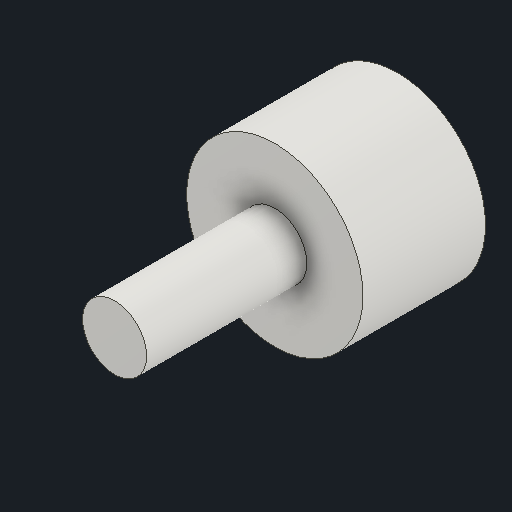
# Autodesk Inventor part: Flat Pulley1
Saved by Autodesk Inventor 2024.2 (Build 282272000, 272)
## iProperties
CustomPartVersion: 1
Created: 2024-03-22
Part Number: Flat Pulley1
Material: Steel
Document SubType Name: Modeling
Designer: LightStore
Density: 7.85 g/cm^3
Appearance: Steel
d3: 0.000 mm
d4: 0.000 mm
Author: LightStore
Autodesk Inventor part; units mm, degrees
ref_plane "YZ Plane" through (0, 0, 0) normal (1, 0, 0) x (0, 1, 0)
ref_plane "XZ Plane" through (0, 0, 0) normal (0, 1, 0) x (-1, 0, 0)
ref_plane "XY Plane" through (0, 0, 0) normal (0, 0, 1) x (1, 0, 0)
sketch "Main Sketch" plane through (0, 0, 0) normal (0, 0, 1) x (1, 0, 0)
  circle A0 centre (0, 0) radius 11
  dimension "d0" = 22
  constraints: 1 centre point, 1 coincident
  measures "d0" diameter of A0
extrude "Pulley" add sketch "Main Sketch" along normal mid plane 15.3
sketch "Sketch2" plane through (0, 0, 7.65) normal (0, 0, 1) x (1, 0, 0)
  circle A0 centre (0, 0) radius 11 projected
  circle A1 centre (0, 0) radius 4
  dimension "d5" = 8
  constraints: 1 centre point, 1 coincident
  measures "d5" diameter of A1
extrude "Extrusion2" add sketch "Sketch2" along normal blind 20 contours A1
equation "\"d0\" = da_D"
equation "\"d1\" = da_B"
equation "\"da_D\" = 22"
equation "\"da_B\" = 15.3"
body "Solid1"
